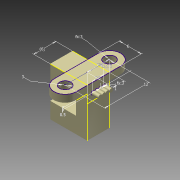
# Autodesk Inventor part: InkrementalisOptikaiErzekelo
Saved by Autodesk Inventor 2015 (Build 190159000, 159)
## iProperties
Created: 2014-11-05
Part Number: InkrementalisOptikaiErzekelo
Material: Nylon 6/6
Document SubType Name: Modeling
Designer: laca
Density: 1.13 g/cm^3
Appearance: Nylon 6
Mass: 0.79615 g
Surface Area: 7.60139 cm^2
Volume: 0.704558 cm^3
Author: laca
Autodesk Inventor part; units mm, degrees
ref_plane "YZ Plane" through (0, 0, 0) normal (1, 0, 0) x (0, 1, 0)
ref_plane "XZ Plane" through (0, 0, 0) normal (0, 1, 0) x (-1, 0, 0)
ref_plane "XY Plane" through (0, 0, 0) normal (0, 0, 1) x (1, 0, 0)
sketch "Sketch2" plane through (0, 0, 0) normal (0, 1, 0) x (-1, 0, 0)
  line L0 (0, 0) -> (10, 0)
  line L1 (10, 0) -> (10, -13)
  line L2 (10, -13) -> (0, -13)
  line L3 (0, -13) -> (0, 0)
  line L4 (10, -4.3333) -> (3, -4.3333)
  line L5 (3, -4.3333) -> (3, -8.6667)
  line L6 (3, -8.6667) -> (10, -8.6667)
  line L7 (10, -8.6667) -> (10, -4.3333)
  dimension "d4" = 13
  dimension "d5" = 10
  dimension "d6" = 4.3333
  dimension "d7" = 7
  dimension "d8" = 4.3333
  constraints: 16 end point, 4 parallel, 2 horizontal, 2 perpendicular, 1 point on line
  measures "d4" distance of L2.end L0.start
  measures "d5" distance of L0.start L0.end
  measures "d6" distance between parallel lines of L0 L4
  measures "d7" distance of L4.start L4.end
  measures "d8" distance of L4.end L5.end
extrude "Extrusion2" add sketch "Sketch2" along normal blind 6 contours L0 L1 L4 L5 L6 L2 L3
sketch "Sketch3" plane through (-10, 0, 0) normal (0, 0, 1) x (1, 0, 0)
  line L0 (7, 9) -> (7, -3) construction
  line L1 (4, 9) -> (4, -3)
  line L2 (10, -3) -> (10, 9)
  arc A0 (10, 9) -> (4, 9) centre (7, 9) ccw
  arc A1 (4, -3) -> (10, -3) centre (7, -3) ccw
  circle A2 centre (7, 9) radius 1.5
  circle A3 centre (7, -3) radius 1.5
  line L3 (10, 0) -> (10, 6) projected
  line L4 (0, 6) -> (10, 6) projected
  line L5 (0, 0) -> (10, 0) projected
  point P0 (7, 3)
  dimension "d11" = 12
  dimension "d12" = 6
  dimension "d13" = 3
  dimension "d14" = 3
  dimension "d15" = 3
  dimension "d16" = 6
  constraints: 8 end point, 4 centre point, 4 point on circle, 4 tangent, 2 coincident, 1 collinear, 1 midpoint, 1 parallel, 1 vertical
  measures "d11" distance of L0.start L0.end
  measures "d12" distance between parallel lines of L2 L1
  measures "d13" diameter of A3
  measures "d14" diameter of A2
  measures "d15" distance from line of point (7, 3) L4
  measures "d16" distance between parallel lines of L5 L4
extrude "Extrusion3" add sketch "Sketch3" against normal blind 2
sketch "Sketch4" plane through (0, 0, -13) normal (1, 0, 0) x (0, 0, -1)
  circle A0 centre (-10.5, 4.5) radius 0.5
  line L0 (-8.6667, 0) -> (-8.6667, 6) projected
  line L1 (-8.6667, 5.6316) -> (-8.6667, 4.1699)
  circle A1 centre (-10.5, 3.5) radius 0.5
  circle A2 centre (-10.5, 2.5) radius 0.5
  circle A3 centre (-10.5, 1.5) radius 0.5
  line L2 (-11, 6) -> (0, 6) projected
  line L3 (-11, 0) -> (0, 0) projected
  line L4 (-11, 0) -> (-11, -3) projected
  point P0 (-13, 0)
  dimension "d19" = 1
  dimension "d22" = 1
  dimension "d27" = 1.5
  dimension "d28" = 3
  dimension "d29" = 6
  dimension "d30" = 0.5
  constraints: 4 centre point, 2 end point, 2 point on line, 1 vertical, 6 other
  measures "d19" diameter of A0
  measures "d22" distance of A0.centre A1.centre
  measures "d27" distance from line of A0.centre L2
  measures "d28" distance of A3.centre A0.centre
  measures "d29" distance between parallel lines of L3 L2
  measures "d30" distance from line of L4 A3.centre
extrude "Extrusion4" add sketch "Sketch4" along normal blind 2
equation "\"d6\" = 0.333333 * d4"
equation "\"d8\" = 0.333333 * d4"
equation "\"d14\" = d13"
equation "\"d15\" = 0.5 * d16"
equation "\"d27\" = -0.5 * d28 + 0.5 * d29"
body "Solid2"
